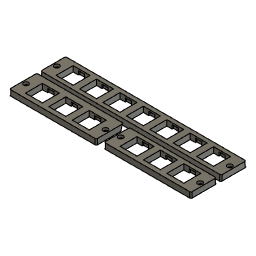
chiron-r7-v21 (Autodesk Fusion 360 archive; units mm, degrees)
design "Chiron Attempt 7 Plates"
Autodesk Fusion 360 part; units mm, degrees
sketch "Sketch1" plane through (0, 0, 0) normal (0, 1, 0) x (1, 0, 0) in component "3 Hole Plate Down"
  line L0 (6.9, -6.9) -> (-6.9, -6.9)
  line L1 (-6.9, -6.9) -> (-6.9, 6.9)
  line L2 (-6.9, 6.9) -> (6.9, 6.9)
  line L3 (6.9, 6.9) -> (6.9, -6.9)
  line L4 (6.9, -6.9) -> (-6.9, 6.9) construction
  line L5 (-6.9, -6.9) -> (6.9, 6.9) construction
  line L6 (12.15, -6.9) -> (12.15, 6.9)
  line L7 (12.15, 6.9) -> (25.95, 6.9)
  line L8 (25.95, 6.9) -> (25.95, -6.9)
  line L9 (25.95, -6.9) -> (12.15, -6.9)
  line L10 (31.2, -6.9) -> (31.2, 6.9)
  line L11 (31.2, 6.9) -> (45, 6.9)
  line L12 (45, 6.9) -> (45, -6.9)
  line L13 (45, -6.9) -> (31.2, -6.9)
  line L14 (-6.9, 0) -> (0, 0) construction
  circle A0 centre (-13.25, 0) radius 1
  circle A1 centre (51.35, 0) radius 1
  line L15 (12.15, -6.9) -> (25.95, 6.9) construction
  line L16 (25.95, -6.9) -> (12.15, 6.9) construction
  line L17 (31.2, -6.9) -> (45, 6.9) construction
  line L18 (45, -6.9) -> (31.2, 6.9) construction
  line L19 (2.5, 6.9) -> (-2.5, 6.9)
  line L20 (-2.5, 6.9) -> (-2.5, 7.9)
  line L21 (-2.5, 7.9) -> (2.5, 7.9)
  line L22 (2.5, 7.9) -> (2.5, 6.9)
  line L23 (2.5, 6.9) -> (-2.5, 7.9) construction
  line L24 (-2.5, 6.9) -> (2.5, 7.9) construction
  line L25 (-2.5, -6.9) -> (2.5, -6.9)
  line L26 (2.5, -6.9) -> (2.5, -7.9)
  line L27 (2.5, -7.9) -> (-2.5, -7.9)
  line L28 (-2.5, -7.9) -> (-2.5, -6.9)
  line L29 (-2.5, -6.9) -> (2.5, -7.9) construction
  line L30 (2.5, -6.9) -> (-2.5, -7.9) construction
  line L31 (16.55, -7.9) -> (16.55, -6.9)
  line L32 (16.55, -6.9) -> (21.55, -6.9)
  line L33 (21.55, -7.9) -> (16.55, -7.9)
  line L34 (21.55, -6.9) -> (21.55, -7.9)
  line L35 (16.55, 6.9) -> (16.55, 7.9)
  line L36 (16.55, 7.9) -> (21.55, 7.9)
  line L37 (21.55, 6.9) -> (16.55, 6.9)
  line L38 (21.55, 7.9) -> (21.55, 6.9)
  line L39 (35.6, -7.9) -> (35.6, -6.9)
  line L40 (35.6, -6.9) -> (40.6, -6.9)
  line L41 (40.6, -7.9) -> (35.6, -7.9)
  line L42 (40.6, -6.9) -> (40.6, -7.9)
  line L43 (35.6, 6.9) -> (35.6, 7.9)
  line L44 (35.6, 7.9) -> (40.6, 7.9)
  line L45 (40.6, 6.9) -> (35.6, 6.9)
  line L46 (40.6, 7.9) -> (40.6, 6.9)
  circle A2 centre (-13.25, 0) radius 2
  circle A3 centre (51.35, 0) radius 2
  line L47 (-16.25, 10.525) -> (54.35, 10.525)
  line L48 (54.35, 10.525) -> (54.35, -10.525)
  line L49 (54.35, -10.525) -> (-16.25, -10.525)
  line L50 (-16.25, -10.525) -> (-16.25, 10.525)
  line L51 (9.25, 9.25) -> (-9.25, 9.25) construction
  line L52 (-9.25, 9.25) -> (-9.25, -9.25) construction
  line L53 (-9.25, -9.25) -> (9.25, -9.25) construction
  line L54 (9.25, -9.25) -> (9.25, 9.25) construction
  line L55 (9.25, 9.25) -> (-9.25, -9.25) construction
  line L56 (-9.25, 9.25) -> (9.25, -9.25) construction
  line L57 (9.8, -9.25) -> (28.3, -9.25) construction
  line L58 (28.3, -9.25) -> (28.3, 9.25) construction
  line L59 (28.3, 9.25) -> (9.8, 9.25) construction
  line L60 (9.8, 9.25) -> (9.8, -9.25) construction
  line L61 (28.85, -9.25) -> (47.35, -9.25) construction
  line L62 (47.35, -9.25) -> (47.35, 9.25) construction
  line L63 (47.35, 9.25) -> (28.85, 9.25) construction
  line L64 (28.85, 9.25) -> (28.85, -9.25) construction
  point P0 (19.05, 0)
  point P1 (38.1, 0)
  point P2 (0, 7.4)
  point P3 (0, -7.4)
  dimension "d2" = 13.8
  dimension "d5" = 19.05
  dimension "d6" = 0
  dimension "d11" = 2
  dimension "d20" = 1
  dimension "d21" = 5
  dimension "d35" = 4
  dimension "d40" = 21.05
  dimension "d41" = 3
  dimension "d42" = 3
  dimension "d52" = 18.5
  dimension "d53" = 18.5
  dimension "d54" = 4
  dimension "d55" = 4
  constraint perpendicular L0 L1
  constraint parallel L0 L2
  constraint parallel L1 L3
  constraint horizontal L0
  constraint coincident L4 L14.end
  constraint coincident L5 L14.end
  constraint coincident L14.end origin
  constraint equal L2 L3
  constraint midpoint L1 L14.start
  constraint horizontal L14.end A0.centre
  constraint horizontal L14.end A1.centre
  constraint equal A0 A1
  constraint perpendicular L19 L20
  constraint parallel L19 L21
  constraint parallel L20 L22
  constraint horizontal L19
  constraint coincident L23 P2
  constraint coincident L24 P2
  constraint vertical L14.end P2
  constraint collinear L2 L19
  constraint perpendicular L25 L26
  constraint parallel L25 L27
  constraint parallel L26 L28
  constraint horizontal L25
  constraint coincident L29 P3
  constraint coincident L30 P3
  constraint vertical P2 P3
  constraint equal L21 L25
  constraint equal L20 L28
  constraint collinear L0 L25
  constraint concentric A0 A2
  constraint concentric A1 A3
  constraint equal A2 A3
  constraint horizontal L47
  constraint vertical L48
  constraint horizontal L49
  constraint vertical L50
  constraint symmetric L14 L47 L49
  constraint perpendicular L51 L52
  constraint parallel L51 L53
  constraint parallel L52 L54
  constraint horizontal L51
  constraint coincident L55 L14.end
  constraint coincident L56 L14.end
  measures "d2" distance of L1.end L2.end
  measures "d11" diameter of A0
  measures "d20" distance of L19.end L20.end
  measures "d21" distance of L20.end L21.end
  measures "d35" diameter of A2
  measures "d40" distance of L47 L49
  measures "d41" distance of A0.centre L50
  measures "d42" distance of A1.centre L48
  measures "d52" distance of L52.end L53.end
  measures "d53" distance of L51.end L52.end
  measures "d54" distance of A0.centre L52
  measures "d55" distance of A1.centre L62
extrude "Extrude1" add sketch "Sketch1" along normal blind 4.5 contours L0 L25 L26 L27 L28 | L2 L19 L20 L21 L22 | L9 L31 L32 L33 L34 | L7 L35 L36 L37 L38 | L13 L39 L40 L41 L42 | L11 L43 L44 L45 L46 | A2 | A3 | L47 L48 L49 L50 makes body 1 in component "3 Hole Plate Down"
extrude "Extrude2" cut sketch "Sketch1" against normal up to surface (3.1 mm away) from surface at 3.1 contours L0 L25 L26 L27 L28 | L2 L19 L20 L21 L22 | L9 L31 L32 L33 L34 | L7 L35 L36 L37 L38 | L13 L39 L40 L41 L42 | L11 L43 L44 L45 L46 bodies 1 in component "3 Hole Plate Down"
extrude "Extrude3" cut sketch "Sketch1" against normal blind 2 from surface at 4.5 contours A0 | A1 | A2 | A3 bodies 1 in component "3 Hole Plate Down"
sketch "Sketch1 (2)" plane through (0, 0, 0) normal (0, 1, 0) x (1, 0, 0) in component "7 Hole Plate"
  line L0 (6.9, -6.9) -> (-6.9, -6.9)
  line L1 (-6.9, -6.9) -> (-6.9, 6.9)
  line L2 (-6.9, 6.9) -> (6.9, 6.9)
  line L3 (6.9, 6.9) -> (6.9, -6.9)
  line L4 (6.9, -6.9) -> (-6.9, 6.9) construction
  line L5 (-6.9, -6.9) -> (6.9, 6.9) construction
  line L6 (12.15, -6.9) -> (12.15, 6.9)
  line L7 (12.15, 6.9) -> (25.95, 6.9)
  line L8 (25.95, 6.9) -> (25.95, -6.9)
  line L9 (25.95, -6.9) -> (12.15, -6.9)
  line L10 (31.2, -6.9) -> (31.2, 6.9)
  line L11 (31.2, 6.9) -> (45, 6.9)
  line L12 (45, 6.9) -> (45, -6.9)
  line L13 (45, -6.9) -> (31.2, -6.9)
  line L14 (-6.9, 0) -> (0, 0) construction
  circle A0 centre (-13.25, 0) radius 1
  circle A1 centre (127.55, 0) radius 1
  line L15 (12.15, -6.9) -> (25.95, 6.9) construction
  line L16 (25.95, -6.9) -> (12.15, 6.9) construction
  line L17 (31.2, -6.9) -> (45, 6.9) construction
  line L18 (45, -6.9) -> (31.2, 6.9) construction
  line L19 (2.5, 6.9) -> (-2.5, 6.9)
  line L20 (-2.5, 6.9) -> (-2.5, 7.9)
  line L21 (-2.5, 7.9) -> (2.5, 7.9)
  line L22 (2.5, 7.9) -> (2.5, 6.9)
  line L23 (2.5, 6.9) -> (-2.5, 7.9) construction
  line L24 (-2.5, 6.9) -> (2.5, 7.9) construction
  line L25 (-2.5, -6.9) -> (2.5, -6.9)
  line L26 (2.5, -6.9) -> (2.5, -7.9)
  line L27 (2.5, -7.9) -> (-2.5, -7.9)
  line L28 (-2.5, -7.9) -> (-2.5, -6.9)
  line L29 (-2.5, -6.9) -> (2.5, -7.9) construction
  line L30 (2.5, -6.9) -> (-2.5, -7.9) construction
  line L31 (16.55, -7.9) -> (16.55, -6.9)
  line L32 (16.55, -6.9) -> (21.55, -6.9)
  line L33 (21.55, -7.9) -> (16.55, -7.9)
  line L34 (21.55, -6.9) -> (21.55, -7.9)
  line L35 (16.55, 6.9) -> (16.55, 7.9)
  line L36 (16.55, 7.9) -> (21.55, 7.9)
  line L37 (21.55, 6.9) -> (16.55, 6.9)
  line L38 (21.55, 7.9) -> (21.55, 6.9)
  line L39 (35.6, -7.9) -> (35.6, -6.9)
  line L40 (35.6, -6.9) -> (40.6, -6.9)
  line L41 (40.6, -7.9) -> (35.6, -7.9)
  line L42 (40.6, -6.9) -> (40.6, -7.9)
  line L43 (35.6, 6.9) -> (35.6, 7.9)
  line L44 (35.6, 7.9) -> (40.6, 7.9)
  line L45 (40.6, 6.9) -> (35.6, 6.9)
  line L46 (40.6, 7.9) -> (40.6, 6.9)
  line L47 (50.25, -6.9) -> (50.25, 6.9)
  line L48 (50.25, 6.9) -> (64.05, 6.9)
  line L49 (64.05, 6.9) -> (64.05, -6.9)
  line L50 (64.05, -6.9) -> (50.25, -6.9)
  line L51 (50.25, -6.9) -> (64.05, 6.9) construction
  line L52 (64.05, -6.9) -> (50.25, 6.9) construction
  line L53 (54.65, -7.9) -> (54.65, -6.9)
  line L54 (54.65, -6.9) -> (59.65, -6.9)
  line L55 (59.65, -7.9) -> (54.65, -7.9)
  line L56 (59.65, -6.9) -> (59.65, -7.9)
  line L57 (54.65, 6.9) -> (54.65, 7.9)
  line L58 (54.65, 7.9) -> (59.65, 7.9)
  line L59 (59.65, 6.9) -> (54.65, 6.9)
  line L60 (59.65, 7.9) -> (59.65, 6.9)
  line L61 (69.3, -6.9) -> (69.3, 6.9)
  line L62 (69.3, 6.9) -> (83.1, 6.9)
  line L63 (83.1, 6.9) -> (83.1, -6.9)
  line L64 (83.1, -6.9) -> (69.3, -6.9)
  line L65 (69.3, -6.9) -> (83.1, 6.9) construction
  line L66 (83.1, -6.9) -> (69.3, 6.9) construction
  line L67 (73.7, -7.9) -> (73.7, -6.9)
  line L68 (73.7, -6.9) -> (78.7, -6.9)
  line L69 (78.7, -7.9) -> (73.7, -7.9)
  line L70 (78.7, -6.9) -> (78.7, -7.9)
  line L71 (73.7, 6.9) -> (73.7, 7.9)
  line L72 (73.7, 7.9) -> (78.7, 7.9)
  line L73 (78.7, 6.9) -> (73.7, 6.9)
  line L74 (78.7, 7.9) -> (78.7, 6.9)
  line L75 (88.35, -6.9) -> (88.35, 6.9)
  line L76 (88.35, 6.9) -> (102.15, 6.9)
  line L77 (102.15, 6.9) -> (102.15, -6.9)
  line L78 (102.15, -6.9) -> (88.35, -6.9)
  line L79 (88.35, -6.9) -> (102.15, 6.9) construction
  line L80 (102.15, -6.9) -> (88.35, 6.9) construction
  line L81 (92.75, -7.9) -> (92.75, -6.9)
  line L82 (92.75, -6.9) -> (97.75, -6.9)
  line L83 (97.75, -7.9) -> (92.75, -7.9)
  line L84 (97.75, -6.9) -> (97.75, -7.9)
  line L85 (92.75, 6.9) -> (92.75, 7.9)
  line L86 (92.75, 7.9) -> (97.75, 7.9)
  line L87 (97.75, 6.9) -> (92.75, 6.9)
  line L88 (97.75, 7.9) -> (97.75, 6.9)
  line L89 (107.4, -6.9) -> (107.4, 6.9)
  line L90 (107.4, 6.9) -> (121.2, 6.9)
  line L91 (121.2, 6.9) -> (121.2, -6.9)
  line L92 (121.2, -6.9) -> (107.4, -6.9)
  line L93 (107.4, -6.9) -> (121.2, 6.9) construction
  line L94 (121.2, -6.9) -> (107.4, 6.9) construction
  line L95 (111.8, -7.9) -> (111.8, -6.9)
  line L96 (111.8, -6.9) -> (116.8, -6.9)
  line L97 (116.8, -7.9) -> (111.8, -7.9)
  line L98 (116.8, -6.9) -> (116.8, -7.9)
  line L99 (111.8, 6.9) -> (111.8, 7.9)
  line L100 (111.8, 7.9) -> (116.8, 7.9)
  line L101 (116.8, 6.9) -> (111.8, 6.9)
  line L102 (116.8, 7.9) -> (116.8, 6.9)
  circle A2 centre (-13.25, 0) radius 2
  circle A3 centre (127.55, 0) radius 2
  line L103 (-16.25, 10.525) -> (130.55, 10.525)
  line L104 (130.55, 10.525) -> (130.55, -10.525)
  line L105 (130.55, -10.525) -> (-16.25, -10.525)
  line L106 (-16.25, -10.525) -> (-16.25, 10.525)
  line L107 (9.25, -9.25) -> (-9.25, -9.25) construction
  line L108 (-9.25, -9.25) -> (-9.25, 9.25) construction
  line L109 (-9.25, 9.25) -> (9.25, 9.25) construction
  line L110 (9.25, 9.25) -> (9.25, -9.25) construction
  line L111 (9.25, -9.25) -> (-9.25, 9.25) construction
  line L112 (-9.25, -9.25) -> (9.25, 9.25) construction
  line L113 (28.3, 9.25) -> (28.3, -9.25) construction
  line L114 (28.3, -9.25) -> (9.8, -9.25) construction
  line L115 (9.8, -9.25) -> (9.8, 9.25) construction
  line L116 (9.8, 9.25) -> (28.3, 9.25) construction
  line L117 (47.35, 9.25) -> (47.35, -9.25) construction
  line L118 (47.35, -9.25) -> (28.85, -9.25) construction
  line L119 (28.85, -9.25) -> (28.85, 9.25) construction
  line L120 (28.85, 9.25) -> (47.35, 9.25) construction
  line L121 (66.4, 9.25) -> (66.4, -9.25) construction
  line L122 (66.4, -9.25) -> (47.9, -9.25) construction
  line L123 (47.9, -9.25) -> (47.9, 9.25) construction
  line L124 (47.9, 9.25) -> (66.4, 9.25) construction
  line L125 (85.45, 9.25) -> (85.45, -9.25) construction
  line L126 (85.45, -9.25) -> (66.95, -9.25) construction
  line L127 (66.95, -9.25) -> (66.95, 9.25) construction
  line L128 (66.95, 9.25) -> (85.45, 9.25) construction
  line L129 (104.5, 9.25) -> (104.5, -9.25) construction
  line L130 (104.5, -9.25) -> (86, -9.25) construction
  line L131 (86, -9.25) -> (86, 9.25) construction
  line L132 (86, 9.25) -> (104.5, 9.25) construction
  line L133 (123.55, 9.25) -> (123.55, -9.25) construction
  line L134 (123.55, -9.25) -> (105.05, -9.25) construction
  line L135 (105.05, -9.25) -> (105.05, 9.25) construction
  line L136 (105.05, 9.25) -> (123.55, 9.25) construction
  point P0 (19.05, 0)
  point P1 (38.1, 0)
  point P2 (0, 7.4)
  point P3 (0, -7.4)
  point P4 (57.15, 0)
  point P5 (76.2, 0)
  point P6 (95.25, 0)
  point P7 (114.3, 0)
  dimension "d2_1" = 13.8
  dimension "d5_1" = 19.05
  dimension "d6_1" = 0
  dimension "d11_1" = 2
  dimension "d20_1" = 1
  dimension "d21_1" = 5
  dimension "d37" = 4
  dimension "d43" = 3
  dimension "d44" = 3
  dimension "d45" = 21.05
  dimension "d56" = 18.5
  dimension "d57" = 18.5
  dimension "d58" = 4
  dimension "d59" = 4
  constraint perpendicular L0 L1
  constraint parallel L0 L2
  constraint parallel L1 L3
  constraint horizontal L0
  constraint coincident L4 L14.end
  constraint coincident L5 L14.end
  constraint coincident L14.end origin
  constraint equal L2 L3
  constraint midpoint L1 L14.start
  constraint horizontal L14.end A0.centre
  constraint horizontal L14.end A1.centre
  constraint equal A0 A1
  constraint perpendicular L19 L20
  constraint parallel L19 L21
  constraint parallel L20 L22
  constraint horizontal L19
  constraint coincident L23 P2
  constraint coincident L24 P2
  constraint vertical L14.end P2
  constraint collinear L2 L19
  constraint perpendicular L25 L26
  constraint parallel L25 L27
  constraint parallel L26 L28
  constraint horizontal L25
  constraint coincident L29 P3
  constraint coincident L30 P3
  constraint vertical P2 P3
  constraint equal L21 L25
  constraint equal L20 L28
  constraint collinear L0 L25
  constraint concentric A0 A2
  constraint concentric A1 A3
  constraint equal A2 A3
  constraint horizontal L103
  constraint vertical L104
  constraint horizontal L105
  constraint vertical L106
  constraint symmetric L14 L103 L105
  constraint perpendicular L107 L108
  constraint parallel L107 L109
  constraint parallel L108 L110
  constraint horizontal L107
  constraint coincident L111 L14.end
  constraint coincident L112 L14.end
  measures "d2_1" distance of L1.end L2.end
  measures "d11_1" diameter of A0
  measures "d20_1" distance of L19.end L20.end
  measures "d21_1" distance of L20.end L21.end
  measures "d37" diameter of A2
  measures "d43" distance of A0.centre L106
  measures "d44" distance of A1.centre L104
  measures "d45" distance of L103 L105
  measures "d56" distance of L107.end L108.end
  measures "d57" distance of L108.end L109.end
  measures "d58" distance of A0.centre L108
  measures "d59" distance of A1.centre L133
extrude "Extrude1'" add sketch "Sketch1 (2)" along normal blind 4.5 separate body contours L0 L25 L26 L27 L28 | L2 L19 L20 L21 L22 | L9 L31 L32 L33 L34 | L7 L35 L36 L37 L38 | L13 L39 L40 L41 L42 | L11 L43 L44 L45 L46 | L50 L53 L54 L55 L56 | L48 L57 L58 L59 L60 | L64 L67 L68 L69 L70 | L62 L71 L72 L73 L74 | L78 L81 L82 L83 L84 | L76 L85 L86 L87 L88 | L92 L95 L96 L97 L98 | L90 L99 L100 L101 L102 | A2 | A3 | L103 L104 L105 L106 makes body 2 in component "7 Hole Plate"
extrude "Extrude2'" cut sketch "Sketch1 (2)" against normal up to surface (3.1 mm away) from surface at 3.1 contours L0 L25 L26 L27 L28 | L2 L19 L20 L21 L22 | L9 L31 L32 L33 L34 | L7 L35 L36 L37 L38 | L13 L39 L40 L41 L42 | L11 L43 L44 L45 L46 | L50 L53 L54 L55 L56 | L48 L57 L58 L59 L60 | L64 L67 L68 L69 L70 | L62 L71 L72 L73 L74 | L78 L81 L82 L83 L84 | L76 L85 L86 L87 L88 | L92 L95 L96 L97 L98 | L90 L99 L100 L101 L102 bodies 2 in component "7 Hole Plate"
extrude "Extrude3'" cut sketch "Sketch1 (2)" against normal blind 2 from surface at 4.5 contours A0 | A1 | A2 | A3 bodies 2 in component "7 Hole Plate"
draft "Draft1" angle -5 neutral plane through (0, 0, 0) pull (0, -1, 0) 2 faces at (81.6167, 1.5, 10.525) (32.6833, 1.5, -10.525) on bodies 2 in component "7 Hole Plate"
draft "Draft1'" angle 15 neutral plane through (0, 0, 0) pull (0, -1, 0) 1 faces at (7.2833, 1.5, -10.525) on bodies 1 in component "3 Hole Plate Down"
fillet "Fillet1" radius 1 4 edges at (-16.25, 2.25, 10.525) (-16.25, 2.25, -11.1279) (54.35, 2.25, 10.525) (54.35, 2.25, -11.1279) on bodies 1 in component "3 Hole Plate Down"
fillet "Fillet1'" radius 1 4 edges at (130.55, 2.25, -10.3282) (130.55, 2.25, 10.3282) (-16.25, 2.25, 10.3282) (-16.25, 2.25, -10.3282) on bodies 2 in component "7 Hole Plate"
sketch "Sketch1 (3)" plane through (0, 0, 0) normal (0, 1, 0) x (1, 0, 0) in component "3 Hole Plate Up"
  line L0 (6.9, -6.9) -> (-6.9, -6.9)
  line L1 (-6.9, -6.9) -> (-6.9, 6.9)
  line L2 (-6.9, 6.9) -> (6.9, 6.9)
  line L3 (6.9, 6.9) -> (6.9, -6.9)
  line L4 (6.9, -6.9) -> (-6.9, 6.9) construction
  line L5 (-6.9, -6.9) -> (6.9, 6.9) construction
  line L6 (12.15, -6.9) -> (12.15, 6.9)
  line L7 (12.15, 6.9) -> (25.95, 6.9)
  line L8 (25.95, 6.9) -> (25.95, -6.9)
  line L9 (25.95, -6.9) -> (12.15, -6.9)
  line L10 (31.2, -6.9) -> (31.2, 6.9)
  line L11 (31.2, 6.9) -> (45, 6.9)
  line L12 (45, 6.9) -> (45, -6.9)
  line L13 (45, -6.9) -> (31.2, -6.9)
  line L14 (-6.9, 0) -> (0, 0) construction
  circle A0 centre (-13.25, 0) radius 1
  circle A1 centre (51.35, 0) radius 1
  line L15 (12.15, -6.9) -> (25.95, 6.9) construction
  line L16 (25.95, -6.9) -> (12.15, 6.9) construction
  line L17 (31.2, -6.9) -> (45, 6.9) construction
  line L18 (45, -6.9) -> (31.2, 6.9) construction
  line L19 (2.5, 6.9) -> (-2.5, 6.9)
  line L20 (-2.5, 6.9) -> (-2.5, 7.9)
  line L21 (-2.5, 7.9) -> (2.5, 7.9)
  line L22 (2.5, 7.9) -> (2.5, 6.9)
  line L23 (2.5, 6.9) -> (-2.5, 7.9) construction
  line L24 (-2.5, 6.9) -> (2.5, 7.9) construction
  line L25 (-2.5, -6.9) -> (2.5, -6.9)
  line L26 (2.5, -6.9) -> (2.5, -7.9)
  line L27 (2.5, -7.9) -> (-2.5, -7.9)
  line L28 (-2.5, -7.9) -> (-2.5, -6.9)
  line L29 (-2.5, -6.9) -> (2.5, -7.9) construction
  line L30 (2.5, -6.9) -> (-2.5, -7.9) construction
  line L31 (16.55, -7.9) -> (16.55, -6.9)
  line L32 (16.55, -6.9) -> (21.55, -6.9)
  line L33 (21.55, -7.9) -> (16.55, -7.9)
  line L34 (21.55, -6.9) -> (21.55, -7.9)
  line L35 (16.55, 6.9) -> (16.55, 7.9)
  line L36 (16.55, 7.9) -> (21.55, 7.9)
  line L37 (21.55, 6.9) -> (16.55, 6.9)
  line L38 (21.55, 7.9) -> (21.55, 6.9)
  line L39 (35.6, -7.9) -> (35.6, -6.9)
  line L40 (35.6, -6.9) -> (40.6, -6.9)
  line L41 (40.6, -7.9) -> (35.6, -7.9)
  line L42 (40.6, -6.9) -> (40.6, -7.9)
  line L43 (35.6, 6.9) -> (35.6, 7.9)
  line L44 (35.6, 7.9) -> (40.6, 7.9)
  line L45 (40.6, 6.9) -> (35.6, 6.9)
  line L46 (40.6, 7.9) -> (40.6, 6.9)
  circle A2 centre (-13.25, 0) radius 2
  circle A3 centre (51.35, 0) radius 2
  line L47 (-16.25, 10.525) -> (54.35, 10.525)
  line L48 (54.35, 10.525) -> (54.35, -10.525)
  line L49 (54.35, -10.525) -> (-16.25, -10.525)
  line L50 (-16.25, -10.525) -> (-16.25, 10.525)
  line L51 (6.9, 6.9) -> (-6.9, 6.9)
  line L52 (-6.9, 6.9) -> (-6.9, -6.9)
  line L53 (-6.9, -6.9) -> (6.9, -6.9)
  line L54 (6.9, -6.9) -> (6.9, 6.9)
  line L55 (6.9, 6.9) -> (-6.9, -6.9) construction
  line L56 (-6.9, 6.9) -> (6.9, -6.9) construction
  line L57 (9.25, 9.25) -> (-9.25, 9.25) construction
  line L58 (-9.25, 9.25) -> (-9.25, -9.25) construction
  line L59 (-9.25, -9.25) -> (9.25, -9.25) construction
  line L60 (9.25, -9.25) -> (9.25, 9.25) construction
  line L61 (9.25, 9.25) -> (-9.25, -9.25) construction
  line L62 (-9.25, 9.25) -> (9.25, -9.25) construction
  line L63 (9.8, -9.25) -> (28.3, -9.25) construction
  line L64 (28.3, -9.25) -> (28.3, 9.25) construction
  line L65 (28.3, 9.25) -> (9.8, 9.25) construction
  line L66 (9.8, 9.25) -> (9.8, -9.25) construction
  line L67 (28.85, -9.25) -> (47.35, -9.25) construction
  line L68 (47.35, -9.25) -> (47.35, 9.25) construction
  line L69 (47.35, 9.25) -> (28.85, 9.25) construction
  line L70 (28.85, 9.25) -> (28.85, -9.25) construction
  point P0 (19.05, 0)
  point P1 (38.1, 0)
  point P2 (0, 7.4)
  point P3 (0, -7.4)
  dimension "d2_2" = 13.8
  dimension "d5_2" = 19.05
  dimension "d6_2" = 0
  dimension "d11_2" = 2
  dimension "d20_2" = 1
  dimension "d21_2" = 5
  dimension "d35_1" = 4
  dimension "d40_1" = 21.05
  dimension "d41_1" = 3
  dimension "d42_1" = 3
  dimension "d60" = 18.5
  dimension "d61" = 18.5
  dimension "d62" = 4
  dimension "d63" = 4
  constraint perpendicular L0 L1
  constraint parallel L0 L2
  constraint parallel L1 L3
  constraint horizontal L0
  constraint coincident L4 L14.end
  constraint coincident L5 L14.end
  constraint coincident L14.end origin
  constraint equal L2 L3
  constraint midpoint L1 L14.start
  constraint horizontal L14.end A0.centre
  constraint horizontal L14.end A1.centre
  constraint equal A0 A1
  constraint perpendicular L19 L20
  constraint parallel L19 L21
  constraint parallel L20 L22
  constraint horizontal L19
  constraint coincident L23 P2
  constraint coincident L24 P2
  constraint vertical L14.end P2
  constraint collinear L2 L19
  constraint perpendicular L25 L26
  constraint parallel L25 L27
  constraint parallel L26 L28
  constraint horizontal L25
  constraint coincident L29 P3
  constraint coincident L30 P3
  constraint vertical P2 P3
  constraint equal L21 L25
  constraint equal L20 L28
  constraint collinear L0 L25
  constraint concentric A0 A2
  constraint concentric A1 A3
  constraint equal A2 A3
  constraint horizontal L47
  constraint vertical L48
  constraint horizontal L49
  constraint vertical L50
  constraint symmetric L14 L47 L49
  constraint perpendicular L51 L52
  constraint parallel L51 L53
  constraint parallel L52 L54
  constraint horizontal L51
  constraint coincident L55 L14.end
  constraint coincident L56 L14.end
  constraint perpendicular L57 L58
  constraint parallel L57 L59
  constraint parallel L58 L60
  constraint horizontal L57
  constraint coincident L61 L14.end
  constraint coincident L62 L14.end
  measures "d2_2" distance of L1.end L2.end
  measures "d11_2" diameter of A0
  measures "d20_2" distance of L19.end L20.end
  measures "d21_2" distance of L20.end L21.end
  measures "d35_1" diameter of A2
  measures "d40_1" distance of L47 L49
  measures "d41_1" distance of A0.centre L50
  measures "d42_1" distance of A1.centre L48
  measures "d60" distance of L58.end L59.end
  measures "d61" distance of L57.end L58.end
  measures "d62" distance of A0.centre L58
  measures "d63" distance of A1.centre L68
extrude "Extrude1''" add sketch "Sketch1 (3)" along normal blind 4.5 separate body contours L0 L25 L26 L27 L28 L53 | L2 L19 L20 L21 L22 L51 | L9 L31 L32 L33 L34 | L7 L35 L36 L37 L38 | L13 L39 L40 L41 L42 | L11 L43 L44 L45 L46 | A2 | A3 | L47 L48 L49 L50 makes body 3 in component "3 Hole Plate Up"
extrude "Extrude2''" cut sketch "Sketch1 (3)" against normal up to surface (3.1 mm away) from surface at 3.1 contours L0 L25 L26 L27 L28 L53 | L2 L19 L20 L21 L22 L51 | L9 L31 L32 L33 L34 | L7 L35 L36 L37 L38 | L13 L39 L40 L41 L42 | L11 L43 L44 L45 L46 bodies 3 in component "3 Hole Plate Up"
extrude "Extrude3''" cut sketch "Sketch1 (3)" against normal blind 2 from surface at 4.5 contours A0 | A1 | A2 | A3 bodies 3 in component "3 Hole Plate Up"
draft "Draft1''" angle -5 neutral plane through (0, 0, 0) pull (0, -1, 0) 1 faces at (7.2833, 1.5, -10.525) on bodies 3 in component "3 Hole Plate Up"
fillet "Fillet1''" radius 1 4 edges at (-16.25, 2.25, 10.525) (-16.25, 2.25, -10.3282) (54.35, 2.25, 10.525) (54.35, 2.25, -10.3282) on bodies 3 in component "3 Hole Plate Up"
component "3 Hole Plate Down" placed x (1, 0, 0) y (0, 1, 0) z (0, 0, 1) at (0, 0, 25)
component "7 Hole Plate" placed x (1, 0, 0) y (0, 1, 0) z (0, 0, 1) at (0, 0, 0)
component "3 Hole Plate Up" placed x (1, 0, 0) y (0, 1, 0) z (0, 0, 1) at (76, 0, 24)
